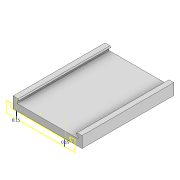
# Autodesk Inventor part: Intan_holder_test
Saved by Autodesk Inventor 2020 (Build 240168000, 168)
## iProperties
Created: 2020-07-20
Part Number: Intan_holder_test
Material: Generic
Document SubType Name: Modeling
Designer: Daniel
Density: 1 g/cm^3
Appearance: Default
Author: Daniel
Autodesk Inventor part; units mm, degrees
ref_plane "YZ Plane" through (0, 0, 0) normal (1, 0, 0) x (0, 1, 0)
ref_plane "XZ Plane" through (0, 0, 0) normal (0, 1, 0) x (-1, 0, 0)
ref_plane "XY Plane" through (0, 0, 0) normal (0, 0, 1) x (1, 0, 0)
sketch "Sketch1" plane through (0, 0, 0) normal (0, 0, 1) x (1, 0, 0)
  line L0 (-9.5, -5) -> (9.5, -5)
  line L1 (9.5, -5) -> (9.5, 5)
  line L2 (9.5, 5) -> (-9.5, 5)
  line L3 (-9.5, 5) -> (-9.5, -5)
  line L4 (-9.5, -5) -> (9.5, 5) construction
  line L5 (9.5, -5) -> (-9.5, 5) construction
  point P0 (0, 0)
  dimension "d0" = 19
  dimension "d1" = 10
  constraints: 12 end point, 2 midpoint, 2 parallel, 1 horizontal, 1 perpendicular
  measures "d0" distance of L0.start L0.end
  measures "d1" distance of L1.end L0.end
extrude "Extrusion1" add sketch "Sketch1" along normal blind 30.18
shell "Shell1" thickness 2 removed faces 1 at (3.1667, -1.6667, 30.18)
sketch "Sketch8" plane through (0, 0, 30.18) normal (0, 0, 1) x (1, 0, 0)
  line L0 (-9.5, -5) -> (9.5, -5) construction
  line L1 (9.5, -5) -> (10.5, -5)
  line L2 (10.5, -5) -> (10.5, 5)
  line L3 (10.5, 5) -> (9.5, 5)
  line L4 (9.5, 5) -> (9.5, -5)
  line L5 (-9.5, 5) -> (-9.5, -5) construction
  line L6 (-9.5, -5) -> (-10.5, -5)
  line L7 (-10.5, -5) -> (-10.5, 5)
  line L8 (-10.5, 5) -> (-9.5, 5)
  line L9 (-9.5, 5) -> (-9.5, -5)
  line L10 (9.5, 5) -> (-9.5, 5) construction
  point P0 (0, 0)
  dimension "d40" = 1
  dimension "d41" = 1
  constraints: 16 end point, 4 parallel, 2 horizontal, 2 perpendicular, 1 collinear, 1 point on line
  measures "d40" distance of L3.end L2.end
  measures "d41" distance of L7.end L8.end
extrude "Extrusion7" add sketch "Sketch8" against normal up to surface (30.18 mm away)
sketch "Sketch3" plane through (0, 0, 0) normal (0, 0, 1) x (1, 0, 0)
  line L0 (-7.5, 3) -> (-7.5, -3) construction
  line L1 (-7.5, -3) -> (7.5, -3) construction
  line L2 (7.5, -3) -> (7.5, 3) construction
  line L3 (7.5, 3) -> (1.5, 3) construction
  line L4 (-9, -4.5) -> (-9, 4.5) construction
  line L5 (-9, 4.5) -> (9, 4.5) construction
  line L6 (9, 4.5) -> (9, -4.5) construction
  line L7 (9, -4.5) -> (-9, -4.5) construction
  line L8 (-9, -2.2) -> (-8.7, -1.9)
  line L9 (-8.7, -1.9) -> (-9, -1.6)
  line L10 (-9, -1.6) -> (-10.5, -1.6)
  line L11 (7.5, -3) -> (-7.5, -3) construction
  line L12 (-9, -3) -> (0, -3)
  line L13 (7.5, 3) -> (-7.5, 3) construction
  line L14 (0, 3) -> (0, -3) construction
  line L15 (-7.5, -3) -> (7.5, -3) construction
  line L16 (-9, -2.2) -> (-9.3, -2.5)
  line L17 (-9.3, -2.5) -> (-9.3, -3)
  line L18 (-9.3, -3) -> (-9, -3)
  line L19 (9, -2.2) -> (8.7, -1.9)
  line L20 (8.7, -1.9) -> (9, -1.6)
  line L21 (9, -1.6) -> (10.5, -1.6)
  line L22 (9, -2.2) -> (9.3, -2.5)
  line L23 (9.3, -2.5) -> (9.3, -3)
  line L24 (9.3, -3) -> (9, -3)
  line L25 (9, -3) -> (0, -3)
  line L26 (1.5, 3) -> (1.5, -0.2) projected
  line L27 (1.5, -0.2) -> (-3.5, -0.2) projected
  line L28 (-3.5, -0.2) -> (-3.5, 3) projected
  line L29 (-3.5, 3) -> (-7.5, 3) projected
  line L30 (-10.5, 5) -> (10.5, 5) construction
  line L31 (10.5, 5) -> (10.5, -5) construction
  line L32 (10.5, -5) -> (-10.5, -5) construction
  line L33 (-10.5, -5) -> (-10.5, 5) construction
  point P0 (0, 0)
  dimension "d10" = 1.5
  dimension "d11" = 0.3
  dimension "d12" = 90
  dimension "d13" = 45
  dimension "d14" = 0.3
  dimension "d15" = 0.5
  constraints: 38 end point, 7 symmetric about line, 4 point on line, 3 perpendicular, 2 horizontal, 2 midpoint, 1 collinear, 1 vertical, 3 other
  measures "d10" distance between parallel lines of L0 L4
  measures "d11" distance from line of L4 L8.end
  measures "d12" angle of L9 L8
  measures "d13" angle of L4 L8
  measures "d14" distance between parallel lines of L4 L17
  measures "d15" distance of L16.end L17.end
sketch "Sketch2" plane through (-7.5, 3, 2) normal (0, 0, 1) x (1, 0, 0)
  line L0 (15, 0) -> (0, 0) construction
  line L1 (4, 0) -> (9, 0)
  line L2 (9, 0) -> (9, -3.2)
  line L3 (9, -3.2) -> (4, -3.2)
  line L4 (4, -3.2) -> (4, 0)
  line L5 (15, -6) -> (15, 0) construction
  point P0 (7.5, -3)
  point P1 (15, -8)
  dimension "d5" = 6
  dimension "d6" = 5
  dimension "d7" = 3.2
  constraints: 8 end point, 2 parallel, 1 horizontal, 1 perpendicular, 1 point on line
  measures "d5" distance between parallel lines of L5 L2
  measures "d6" distance between parallel lines of L4 L2
  measures "d7" distance between parallel lines of L0 L3
extrude "Extrusion2" cut sketch "Sketch2" against normal through all
sketch "Sketch6" plane through (-7.5, 3, 30.18) normal (0, -1, 0) x (1, 0, 0)
  line L0 (15, -28.18) -> (9, -28.18) construction
  line L1 (15, -28.18) -> (15, 0) construction
  line L2 (0, 0) -> (15, 0) construction
  line L3 (0, -28.18) -> (0, 0) construction
  line L4 (4, -28.18) -> (0, -28.18) construction
  line L5 (4, -28.18) -> (4, -30.18) construction
  line L6 (9, -30.18) -> (4, -30.18) construction
  line L7 (9, -28.18) -> (9, -30.18) construction
  line L8 (11.76, -25.02) -> (11.76, -25.62) construction
  line L9 (10.49, -25.02) -> (10.49, -25.62)
  line L10 (13.03, -25.62) -> (13.03, -25.02)
  arc A0 (13.03, -25.02) -> (10.49, -25.02) centre (11.76, -25.02) ccw
  arc A1 (10.49, -25.62) -> (13.03, -25.62) centre (11.76, -25.62) ccw
  point P0 (7.5, -30.18)
  point P1 (11.76, -25.32)
  dimension "d24" = 0.6
  dimension "d25" = 2.54
  dimension "d26" = 2.56
  dimension "d27" = 11.76
  constraints: 8 end point, 4 point on circle, 4 tangent, 2 centre point, 1 midpoint, 1 parallel, 1 vertical
  measures "d24" distance of L8.start L8.end
  measures "d25" diameter of A1
  measures "d26" distance from line of L0 L8.end
  measures "d27" distance from line of L3 L8.start
extrude "Extrusion5" cut sketch "Sketch6" against normal through all
surface extrude "ExtrusionSrf1" sketch "Sketch3" along normal up to surface (30.18 mm away) shown no curves L10 L9 L8 L16 L17 L18 L12 L25 L24 L23 L22 L19 L20 L21
split body "Split1" result two bodies by surface "ExtrusionSrf1" first body at (1.2699, 4.5, 22.2358)
thicken "Thicken1" operation cut thickness 0.2 both sides no extend neighbours no toward (0, 1, 0) faces at (-10, -1.6, 10.06) (-8.9, -1.7, 20.12) (-8.8, -2, 20.12) (-9.1, -2.3, 10.06) (-9.3, -2.6667, 10.06) (-9.2, -3, 10.06) (-6, -3, 10.06) (3, -3, 10.06) (9.1, -3, 10.06) (9.3, -2.8333, 10.06) (9.2, -2.4, 20.12) (8.9, -2.1, 10.06) (8.8, -1.8, 10.06) (9.5, -1.6, 10.06)
sketch "Sketch4" plane through (0, 0, 30.18) normal (0, 0, 1) x (1, 0, 0)
  line L0 (-10.5, -1.6) -> (-9, -1.6) projected
  line L1 (9, -1.6) -> (10.5, -1.6) projected
  line L2 (8.7, -1.9) -> (9, -1.6) projected
  line L3 (9.3, -2.5) -> (8.7, -1.9) projected
  line L4 (9.3, -3) -> (9.3, -2.5) projected
  line L5 (9.3, -3) -> (-9.3, -3) projected
  line L6 (-9.3, -2.5) -> (-9.3, -3) projected
  line L7 (-8.7, -1.9) -> (-9.3, -2.5) projected
  line L8 (-9, -1.6) -> (-8.7, -1.9) projected
  line L9 (7.5, 3) -> (7.5, -2.8) construction
  line L10 (-7.5, -2.8) -> (-7.5, 3) construction
  line L11 (-9.3, -3) -> (9.3, -3) construction
  line L12 (7.35, -3) -> (7.35, -5)
  line L13 (-7.35, -3) -> (-7.35, -5)
  line L14 (-10.5, -1.6) -> (-10.5, -5) projected
  line L15 (-10.5, -5) -> (10.5, -5) projected
  line L16 (10.5, -5) -> (10.5, -1.6) projected
  point P0 (0, 0)
  dimension "d30" = 0.15
  dimension "d31" = 0.15
  constraints: 4 end point, 3 point on line, 1 perpendicular
  measures "d30" distance between parallel lines of L13 L10
  measures "d31" distance between parallel lines of L9 L12
extrude "Extrusion3" cut sketch "Sketch4" against normal blind 2.15
sketch "Sketch5" plane through (8.9172, -1.4, 30.18) normal (0, -1, 0) x (1, 0, 0)
  line L0 (-19.4172, -30.18) -> (-19.4172, 0) construction
  line L1 (1.5828, -30.18) -> (1.5828, 0) construction
  line L2 (-19.4172, 0) -> (1.5828, 0)
  line L3 (1.5828, 0) -> (1.5828, -2)
  line L4 (1.5828, -2) -> (-19.4172, -2)
  line L5 (-19.4172, -2) -> (-19.4172, 0)
  line L6 (-1.4172, -28.18) -> (-1.4172, 0) construction
  line L7 (-1.4172, 0) -> (-1.4172, -2)
  line L8 (-16.4172, -28.18) -> (-16.4172, 0) construction
  line L9 (-16.4172, 0) -> (-16.4172, -2)
  point P0 (-8.9172, -30.18)
  dimension "d21" = 2
  constraints: 12 end point, 5 point on line, 2 parallel, 1 horizontal, 1 perpendicular
  measures "d21" distance between parallel lines of L2 L4
extrude "Extrusion4" add sketch "Sketch5" along normal up to surface (3.6 mm away) contours L2 L9 L4 L5 | L2 L3 L4 L7
chamfer "Chamfer1" distance 1 angle 45 4 edges at (-3.5, 1.4, 0) (-1, 3, 0) (1.5, 1.4, 0) (-1, -0.2, 0)
sketch "Sketch10" plane through (0, 0, 0) normal (0, 0, -1) x (-1, 0, 0)
  line L0 (10.5, 5) -> (-10.5, 5) construction
  line L1 (10.5, 5) -> (9, 5)
  line L2 (9, 5) -> (9, 1)
  line L3 (9, 1) -> (10.5, 1)
  line L4 (10.5, 1) -> (10.5, 5)
  line L5 (-10.5, 5) -> (-9, 5)
  line L6 (-9, 5) -> (-9, 1)
  line L7 (-9, 1) -> (-10.5, 1)
  line L8 (-10.5, 1) -> (-10.5, 5)
  point P0 (0, 0)
  dimension "d46" = 1.5
  dimension "d47" = 4
  dimension "d48" = 1.5
  dimension "d49" = 4
  constraints: 16 end point, 4 parallel, 2 horizontal, 2 perpendicular
  measures "d46" distance of L3.end L2.end
  measures "d47" distance of L2.end L1.end
  measures "d48" distance of L6.end L7.end
  measures "d49" distance of L5.end L6.end
extrude "Extrusion9" cut sketch "Sketch10" against normal blind 29.18
chamfer "Chamfer3" distance 1.5 angle 45 2 edges at (-9, 1, 14.59) (9, 1, 14.59)
equation "\"d13\" = 0.5 * d12"
body "Srf1"
body "Solid2"
body "Solid3"
